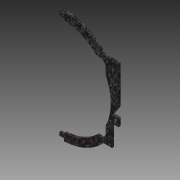
# Autodesk Inventor part: BottomHoop_v1
Saved by Autodesk Inventor 2013 (Build 170138000, 138)
## iProperties
Created: 2013-01-17
Part Number: BottomHoop_v1
Material: Concrete
Document SubType Name: Modeling
Designer: motoennies
Density: 1 g/cm^3
Author: motoennies
Autodesk Inventor part; units mm, degrees
ref_plane "YZ Plane" through (0, 0, 0) normal (1, 0, 0) x (0, 1, 0)
ref_plane "XZ Plane" through (0, 0, 0) normal (0, 1, 0) x (-1, 0, 0)
ref_plane "XY Plane" through (0, 0, 0) normal (0, 0, 1) x (1, 0, 0)
sketch "Sketch1" plane through (0, 0, 0) normal (0, 0, 1) x (1, 0, 0)
  arc A0 (6.35, -145.9119) -> (0, 146.05) centre (0, 0) ccw
  line L0 (0, 0) -> (0, 323.4187) construction
  line L1 (0, 0) -> (0, -168.91) construction
  line L2 (6.35, -168.7906) -> (6.35, -145.9119)
  line L3 (6.35, 145.9119) -> (6.35, 168.7906)
  line L4 (0, -146.05) -> (0, -151.13)
  line L5 (0, -151.13) -> (6.35, -151.13)
  line L6 (6.35, -151.13) -> (-7.62, -151.13)
  line L7 (-7.62, -151.13) -> (-7.62, -161.29)
  line L8 (-7.62, -161.29) -> (6.35, -161.29)
  line L9 (0, 146.05) -> (0, 151.13)
  line L10 (0, 151.13) -> (6.35, 151.13)
  line L11 (6.35, 151.13) -> (-7.62, 151.13)
  line L12 (-7.62, 151.13) -> (-7.62, 161.29)
  line L13 (-7.62, 161.29) -> (6.35, 161.29)
  line L14 (168.91, 0) -> (168.91, -114.3)
  line L15 (168.91, -114.3) -> (124.3628, -114.3)
  arc A1 (124.3628, 114.3) -> (6.35, 168.7906) centre (0, 0) ccw
  arc A2 (6.35, -168.7906) -> (124.3628, -114.3) centre (0, 0) ccw
  line L16 (0, 0) -> (-12.7, 0)
  line L17 (-12.7, 0) -> (324.8812, 0) construction
  line L18 (168.91, 0) -> (168.91, 114.3)
  line L19 (168.91, 114.3) -> (124.3628, 114.3)
  line L20 (146.05, 0) -> (146.05, 82.55) construction
  line L21 (146.05, 82.55) -> (120.4828, 82.55) construction
  line L22 (146.05, 0) -> (146.05, -82.55) construction
  line L23 (146.05, -82.55) -> (120.4828, -82.55) construction
  line L24 (146.05, -82.55) -> (120.4828, -82.55) construction
  line L25 (130.6254, -90.1931) -> (121.4538, -102.3643)
  line L26 (121.4538, -102.3643) -> (104.1737, -102.3643)
  line L27 (130.6254, 90.1931) -> (121.447, 102.3733)
  line L28 (104.1648, 102.3733) -> (121.447, 102.3733)
  line L29 (130.6254, 90.1931) -> (130.6254, 65.3268)
  line L30 (130.6254, -90.1931) -> (130.6254, -65.3268)
  dimension "d0" = 292.1
  dimension "d7" = 6.35
  dimension "d8" = 6.35
  dimension "d9" = 5.08
  dimension "d10" = 13.97
  dimension "d11" = 10.16
  dimension "d12" = 5.08
  dimension "d13" = 13.97
  dimension "d14" = 10.16
  dimension "d16" = 5.2181
  dimension "d35" = 12.7
  dimension "d38" = 114.3
  dimension "d57" = 114.3
  dimension "d58" = 82.55
  dimension "d59" = 82.55
  dimension "d60" = 12.7
  dimension "d63" = 12.7
  dimension "d66" = 127
  constraints: 62 end point, 15 perpendicular, 10 point on line, 5 collinear, 5 vertical, 4 point on circle, 3 horizontal, 3 parallel, 2 centre point, 2 coincident, 2 tangent, 14 other
  measures "d7" distance between parallel lines of L2 L1
  measures "d8" distance between parallel lines of L0 L3
  measures "d9" distance of L4.start L4.end
  measures "d10" distance of L5.end L6.end
  measures "d11" distance of L6.end L7.end
  measures "d12" distance of L9.start L9.end
  measures "d13" distance of L10.end L11.end
  measures "d14" distance of L11.end L12.end
  measures "d16" distance from line of L5 L2.end
  measures "d35" distance of L0.start L16.end
  measures "d38" distance of L14.start L18.end
  measures "d57" distance between parallel lines of L17 L15
  measures "d58" distance of L20.start L20.end
  measures "d59" distance of L20.start L22.end
  measures "d60" distance of L23.end L25.start
  measures "d63" distance of L21.end L27.start
  measures "d66" angle of L28 L27
extrude "Extrusion2" add sketch "Sketch1" along normal blind 6.35 contours A0 L26 L25 L30 L29 L27 L28 L3 A1 L19 L18 L14 L15 A2 L2 | L2 L8 L7 L6 L5 | L10 L11 L12 L13 L3
sketch "Sketch3" plane through (0, 0, 6.35) normal (0, 0, 1) x (1, 0, 0)
  line L0 (124.3628, -114.3) -> (168.91, -114.3) projected
  line L1 (168.91, -114.3) -> (168.91, 114.3) projected
  line L2 (168.91, -114.3) -> (168.91, -43.2308) construction
  line L3 (168.91, -43.2308) -> (163.83, -43.2308) construction
  line L4 (163.83, -43.2308) -> (153.67, -43.2308)
  line L5 (153.67, -43.2308) -> (153.67, -33.7058)
  line L6 (153.67, -33.7058) -> (163.83, -33.7058)
  line L7 (163.83, -33.7058) -> (163.83, -43.2308)
  line L8 (168.91, -50.8) -> (149.86, -50.8)
  line L9 (149.86, -50.8) -> (149.86, -76.2)
  line L10 (149.86, -76.2) -> (149.86, -114.3)
  line L11 (149.86, -114.3) -> (168.91, -114.3)
  line L12 (168.91, -50.8) -> (168.91, -114.3)
  line L13 (168.91, -27.0751) -> (151.13, -27.0751)
  line L14 (151.13, -27.0751) -> (168.91, 0)
  line L15 (168.91, 0) -> (168.91, -27.0751)
  dimension "d46" = 71.0692
  dimension "d47" = 5.08
  dimension "d48" = 10.16
  dimension "d49" = 9.525
  dimension "d50" = 10.16
  dimension "d51" = 19.05
  dimension "d52" = 63.5
  dimension "d53" = 25.4
  dimension "d54" = 17.78
  constraints: 28 end point, 9 perpendicular, 4 point on line, 1 collinear, 1 midpoint, 1 parallel
  measures "d46" distance of L0.end L2.end
  measures "d47" distance of L2.end L3.end
  measures "d48" distance of L3.end L4.end
  measures "d49" distance of L4.end L5.end
  measures "d50" distance of L5.end L6.end
  measures "d51" distance of L8.start L8.end
  measures "d52" distance between parallel lines of L0 L8
  measures "d53" distance of L8.end L9.end
  measures "d54" distance of L13.start L13.end
extrude "Extrusion5" cut sketch "Sketch3" against normal blind 25.4
body "Solid2"
